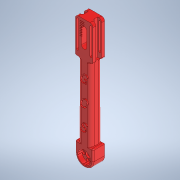
# Autodesk Inventor part: Eslabon1
Saved by Autodesk Inventor 2021 (Build 250183000, 183)
## iProperties
Created: 2022-10-26
Part Number: Eslabon1
Material: Generic
Document SubType Name: Modeling
Designer: USUARIO
Density: 1 g/cm^3
Appearance: Light Red
Mass: 84.0555 g
Surface Area: 248.63 cm^2
Volume: 84.0555 cm^3
Author: USUARIO
Autodesk Inventor part; units mm, degrees
ref_plane "YZ Plane" through (0, 0, 0) normal (1, 0, 0) x (0, 1, 0)
ref_plane "XZ Plane" through (0, 0, 0) normal (0, 1, 0) x (-1, 0, 0)
ref_plane "XY Plane" through (0, 0, 0) normal (0, 0, 1) x (1, 0, 0)
sketch "Sketch1" plane through (0, 0, 0) normal (0, 0, 1) x (1, 0, 0)
  line L0 (0, 0) -> (0, 190) construction
  line L1 (15, 0) -> (15, 190)
  line L2 (-15, 190) -> (-15, 0)
  arc A0 (-15, 0) -> (15, 0) centre (0, 0) ccw
  arc A1 (15, 190) -> (-15, 190) centre (0, 190) ccw
  line L3 (-15, 175) -> (15, 175)
  line L4 (15, 175) -> (15, 200)
  line L5 (10, 205) -> (-10, 205)
  line L6 (-15, 200) -> (-15, 175)
  line L7 (-15, 175) -> (15, 205) construction
  line L8 (15, 175) -> (-15, 205) construction
  arc A2 (-10, 205) -> (-15, 200) centre (-10, 200) ccw
  arc A3 (15, 200) -> (10, 205) centre (10, 200) ccw
  point P0 (0, 95)
  point P1 (0, 205)
  dimension "d0" = 190
  dimension "d1" = 30
  dimension "d48" = 5
  dimension "d49" = 30
  dimension "d50" = 30
  constraints: 20 end point, 8 point on circle, 8 tangent, 4 centre point, 4 point on line, 3 midpoint, 3 parallel, 1 equal radius, 1 horizontal, 1 perpendicular, 1 vertical
  measures "d0" distance of L0.start L0.end
  measures "d1" diameter of A1
  measures "d48" radius of A2
  measures "d49" distance between parallel lines of L6 L4
  measures "d50" distance between parallel lines of L3 L5
extrude "Extrusion1" add sketch "Sketch1" along normal blind 20
sketch "Sketch2" plane through (0, 0, 20) normal (0, 0, 1) x (1, 0, 0)
  arc A0 (15, 185) -> (-15, 185) centre (0, 185) ccw projected
  arc A1 (-15, 0) -> (15, 0) centre (0, 0) ccw projected
  circle A2 centre (0, 0) radius 11
  dimension "d4" = 22
  constraints: 1 centre point, 1 coincident
  measures "d4" diameter of A2
extrude "Extrusion2" cut sketch "Sketch2" against normal blind 7
sketch "Sketch3" plane through (0, 0, 0) normal (0, 0, -1) x (-1, 0, 0)
  circle A0 centre (0, 0) radius 11 projected
  circle A1 centre (0, 0) radius 11
  circle A2 centre (0, 0) radius 2
  circle A3 centre (0, 0) radius 8 construction
  arc A4 (15, 185) -> (-15, 185) centre (0, 185) ccw construction
  circle A5 centre (0, 8) radius 1.5
  line L0 (0, 0) -> (0, 12.8172) construction
  circle A6 centre (-8, 0) radius 1.5
  circle A7 centre (0, -8) radius 1.5
  circle A8 centre (8, 0) radius 1.5
  circle A9 centre (0, 0) radius 5
  dimension "d9" = 16
  dimension "d7" = 22
  dimension "d8" = 4
  dimension "d10" = 3
  dimension "d13" = 360
  dimension "d15" = 10
  constraints: 7 centre point, 4 coincident, 2 end point, 1 point on line, 1 vertical, 1 vertical alignment, 11 other
  measures "d7" diameter of A1
  measures "d8" diameter of A2
  measures "d10" diameter of A5
  measures "d15" diameter of A9
extrude "Extrusion4" cut sketch "Sketch3" against normal through all contours A5 | A6 | A7 | A8
sketch "Sketch4" plane through (0, 0, 13) normal (0, 0, 1) x (1, 0, 0)
  circle A0 centre (-8, 0) radius 1.5 projected
  circle A1 centre (0, 0) radius 2 construction
  circle A2 centre (0, 0) radius 8 construction
  line L0 (-5, 1.7321) -> (-5, -1.7321)
  line L1 (-5, -1.7321) -> (-8, -3.4641)
  line L2 (-8, -3.4641) -> (-11, -1.7321)
  line L3 (-11, -1.7321) -> (-11, 1.7321)
  line L4 (-11, 1.7321) -> (-8, 3.4641)
  line L5 (-8, 3.4641) -> (-5, 1.7321)
  line L6 (-3.4641, -8) -> (-1.7321, -5)
  line L7 (-1.7321, -5) -> (1.7321, -5)
  line L8 (1.7321, -5) -> (3.4641, -8)
  line L9 (3.4641, -8) -> (1.7321, -11)
  line L10 (1.7321, -11) -> (-1.7321, -11)
  line L11 (-1.7321, -11) -> (-3.4641, -8)
  line L12 (8, -3.4641) -> (5, -1.7321)
  line L13 (5, -1.7321) -> (5, 1.7321)
  line L14 (5, 1.7321) -> (8, 3.4641)
  line L15 (8, 3.4641) -> (11, 1.7321)
  line L16 (11, 1.7321) -> (11, -1.7321)
  line L17 (11, -1.7321) -> (8, -3.4641)
  line L18 (3.4641, 8) -> (1.7321, 5)
  line L19 (1.7321, 5) -> (-1.7321, 5)
  line L20 (-1.7321, 5) -> (-3.4641, 8)
  line L21 (-3.4641, 8) -> (-1.7321, 11)
  line L22 (-1.7321, 11) -> (1.7321, 11)
  line L23 (1.7321, 11) -> (3.4641, 8)
  dimension "d20" = 6
  dimension "d23" = 360
  constraints: 48 end point, 3 coincident, 1 horizontal alignment, 1 vertical, 64 other
  measures "d20" distance between parallel lines of L3 L0
extrude "Extrusion5" cut sketch "Sketch4" along normal blind 8.175 and the other way blind 3.5
extrude "Extrusion6" cut sketch "Sketch3" against normal blind 2 contours A0 | A2 | A9
extrude "Extrusion7" cut sketch "Sketch3" against normal through all contours A2
sketch "Sketch5" plane through (0, 0, 13) normal (0, 0, 1) x (1, 0, 0)
  circle A0 centre (0, 0) radius 2 projected
  circle A1 centre (0, 0) radius 4.5
  dimension "d33" = 9
  constraints: 1 centre point, 1 coincident
  measures "d33" diameter of A1
extrude "Extrusion8" cut sketch "Sketch5" against normal blind 3
sketch "Sketch9" plane through (0, 0, 20) normal (0, 0, 1) x (1, 0, 0)
  line L0 (-15, 200) -> (-15, 0) projected
  arc A0 (-15, 0) -> (15, 0) centre (0, 0) ccw projected
  line L1 (15, 0) -> (15, 200) projected
  arc A1 (15, 200) -> (10, 205) centre (10, 200) ccw projected
  line L2 (10, 205) -> (-10, 205) projected
  arc A2 (-10, 205) -> (-15, 200) centre (-10, 200) ccw projected
  line L3 (10.8485, 1.8195) -> (11, 1.7321) projected
  line L4 (11, 1.7321) -> (11, -1.7321) projected
  line L5 (11, -1.7321) -> (10.8485, -1.8195) projected
  arc A3 (1.8195, -10.8485) -> (10.8485, -1.8195) centre (0, 0) ccw projected
  line L6 (1.8195, -10.8485) -> (1.7321, -11) projected
  line L7 (1.7321, -11) -> (-1.7321, -11) projected
  line L8 (-1.7321, -11) -> (-1.8195, -10.8485) projected
  arc A4 (-10.8485, -1.8195) -> (-1.8195, -10.8485) centre (0, 0) ccw projected
  line L9 (-10.8485, -1.8195) -> (-11, -1.7321) projected
  line L10 (-11, -1.7321) -> (-11, 1.7321) projected
  line L11 (-11, 1.7321) -> (-10.8485, 1.8195) projected
  arc A5 (-1.8195, 10.8485) -> (-10.8485, 1.8195) centre (0, 0) ccw projected
  line L12 (-1.8195, 10.8485) -> (-1.7321, 11) projected
  line L13 (-1.7321, 11) -> (1.7321, 11) projected
  line L14 (1.7321, 11) -> (1.8195, 10.8485) projected
  arc A6 (10.8485, 1.8195) -> (1.8195, 10.8485) centre (0, 0) ccw projected
  line L15 (10, 205) -> (-10, 205) projected
  circle A7 centre (0, 0) radius 2 projected
  line L16 (0, 205) -> (0, 0) construction
  line L17 (0, 190) -> (0, 165) construction
  line L18 (-4.5, 190) -> (-4.5, 165)
  line L19 (4.5, 165) -> (4.5, 190)
  arc A8 (4.5, 190) -> (-4.5, 190) centre (0, 190) ccw
  arc A9 (-4.5, 165) -> (4.5, 165) centre (0, 165) ccw
  point P0 (0, 177.5)
  dimension "d51" = 25
  dimension "d52" = 9
  dimension "d53" = 190
  constraints: 10 end point, 4 point on circle, 4 tangent, 2 centre point, 2 midpoint, 2 point on line, 1 parallel, 1 vertical
  measures "d51" distance of L17.start L17.end
  measures "d52" diameter of A9
  measures "d53" distance of point (0, 0) L17.start
extrude "Extrusion11" cut sketch "Sketch9" against normal through all contours A8 L19 A9 L18
sketch "Sketch10" plane through (-10, 205, 0) normal (0, 1, 0) x (1, 0, 0)
  line L0 (14.5, -20) -> (5.5, -20) projected
  line L1 (5.5, -20) -> (14.5, -20) projected
  line L2 (-5, -20) -> (25, -20) projected
  line L3 (25, -20) -> (20, -20) projected
  line L4 (20, -20) -> (0, -20) projected
  line L5 (0, -20) -> (-5, -20) projected
  line L6 (20.8485, -20) -> (21, -20) projected
  line L7 (21, -20) -> (20.8485, -20) projected
  line L8 (20.8485, -20) -> (11.8195, -20) projected
  line L9 (11.8195, -20) -> (11.7321, -20) projected
  line L10 (11.7321, -20) -> (8.2679, -20) projected
  line L11 (8.2679, -20) -> (8.1805, -20) projected
  line L12 (8.1805, -20) -> (-0.8485, -20) projected
  line L13 (-0.8485, -20) -> (-1, -20) projected
  line L14 (-1, -20) -> (-0.8485, -20) projected
  line L15 (-0.8485, -20) -> (8.1805, -20) projected
  line L16 (8.1805, -20) -> (8.2679, -20) projected
  line L17 (8.2679, -20) -> (11.7321, -20) projected
  line L18 (11.7321, -20) -> (11.8195, -20) projected
  line L19 (11.8195, -20) -> (20.8485, -20) projected
  line L20 (25, 0) -> (25, -20) projected
  line L21 (25, 0) -> (25, -20) projected
  line L22 (14.5, 0) -> (5.5, 0) projected
  line L23 (5.5, 0) -> (14.5, 0) projected
  line L24 (-1, 0) -> (21, 0) projected
  line L25 (0, 0) -> (-5, 0) projected
  line L26 (20, 0) -> (0, 0) projected
  line L27 (25, 0) -> (20, 0) projected
  line L28 (-5, 0) -> (25, 0) projected
  line L29 (-5, 0) -> (-5, -20) projected
  line L30 (-5, 0) -> (-5, -20) projected
  line L31 (-5, 0) -> (-5, -20) projected
  line L32 (-5, -5) -> (2, -5)
  line L33 (2, -5) -> (2, -15)
  line L34 (2, -15) -> (-5, -15)
  line L35 (-5, -15) -> (-5, -5)
  line L36 (10, 0) -> (10, -20)
  line L37 (-5, -20) -> (25, -20) projected
  line L38 (25, -5) -> (18, -5)
  line L39 (18, -5) -> (18, -15)
  line L40 (18, -15) -> (25, -15)
  line L41 (25, -15) -> (25, -5)
  point P0 (-5, -15)
  dimension "d56" = 5
  dimension "d57" = 5
  dimension "d58" = 7
  constraints: 18 end point, 4 symmetric about line, 2 parallel, 1 horizontal, 1 perpendicular, 4 other
  measures "d56" distance between parallel lines of L28 L32
  measures "d57" distance between parallel lines of L2 L34
  measures "d58" distance of L33.end L34.end
extrude "Extrusion12" cut sketch "Sketch10" against normal blind 60 contours L40 L39 L38 L20 | L32 L33 L34 L29
sketch "Sketch11" plane through (0, 0, 0) normal (0, 0, -1) x (-1, 0, 0)
  arc A0 (-10, 205) -> (-15, 200) centre (-10, 200) ccw projected
  line L0 (-15, 145) -> (-15, 200) projected
  line L1 (-15, 145) -> (-8, 145) projected
  line L2 (-8, 205) -> (-8, 145) projected
  line L3 (-10, 205) -> (-8, 205) projected
  arc A1 (15, 200) -> (10, 205) centre (10, 200) ccw projected
  line L4 (8, 205) -> (10, 205) projected
  line L5 (8, 205) -> (8, 145) projected
  line L6 (8, 145) -> (15, 145) projected
  line L7 (15, 200) -> (15, 145) projected
  line L8 (-11.5, 145) -> (-11.5, 208.2052) construction
  line L9 (-11.5, 200) -> (-11.5, 155) construction
  line L10 (-13, 200) -> (-13, 155)
  line L11 (-10, 155) -> (-10, 200)
  arc A2 (-10, 200) -> (-13, 200) centre (-11.5, 200) ccw
  arc A3 (-13, 155) -> (-10, 155) centre (-11.5, 155) ccw
  arc A4 (-4.5, 165) -> (4.5, 165) centre (0, 165) ccw projected
  line L12 (4.5, 190) -> (4.5, 165) projected
  line L13 (-4.5, 165) -> (-4.5, 190) construction
  line L14 (-4.5, 177.5) -> (-11.5, 177.5) construction
  line L15 (-10, 205) -> (10, 205) projected
  line L16 (0, 205) -> (0, 150.8166) construction
  line L17 (13, 200) -> (13, 155)
  line L18 (10, 155) -> (10, 200)
  arc A5 (13, 200) -> (10, 200) centre (11.5, 200) ccw
  arc A6 (10, 155) -> (13, 155) centre (11.5, 155) ccw
  point P0 (0, 0)
  dimension "d61" = 3
  dimension "d62" = 45
  dimension "d73" = 23
  constraints: 18 end point, 8 point on circle, 6 symmetric about line, 4 centre point, 4 midpoint, 4 tangent, 2 point on line, 2 vertical, 1 horizontal, 1 parallel, 2 other
  measures "d61" diameter of A3
  measures "d62" distance of L10.start L10.end
  measures "d73" distance of A5.centre L9.start
extrude "Extrusion13" cut sketch "Sketch11" against normal through all contours A2 L11 A3 L10 | L17 A6 L18 A5
fillet "Fillet1" radius 4 2 edges at (8, 175, 15) (-8, 175, 15)
sketch "Sketch12" plane through (0, 0, 20) normal (0, 0, 1) x (1, 0, 0)
  line L0 (-19.28, 124.6729) -> (14.3731, 124.6729) construction
  line L1 (14.3731, 124.6729) -> (14.3731, 20.6875) construction
  line L2 (14.3731, 20.6875) -> (-19.28, 20.6875) construction
  line L3 (-19.28, 20.6875) -> (-19.28, 124.6729) construction
  line L4 (7.1676, 120.3037) -> (4.9576, 119.8084)
  spline S0 degree 2 poles (4.9576, 119.8084) (5.2116, 122.8566) (2.5952, 122.8566) knots 0 0 0 1 1 1
  spline S1 degree 2 poles (2.5952, 122.8566) (0.6138, 122.8566) (-1.0754, 121.1674) knots 0 0 0 1 1 1
  spline S2 degree 2 poles (-1.0754, 121.1674) (-2.6376, 119.6051) (-3.5521, 116.9252) knots 0 0 0 1 1 1
  spline S3 degree 2 poles (-3.5521, 116.9252) (-4.5936, 113.8261) (-3.8569, 112.2766) knots 0 0 0 1 1 1
  spline S4 degree 2 poles (-3.8569, 112.2766) (-3.2346, 110.9684) (-1.4691, 110.9684) knots 0 0 0 1 1 1
  spline S5 degree 2 poles (-1.4691, 110.9684) (0.2709, 110.9684) (1.7188, 112.4544) knots 0 0 0 1 1 1
  spline S6 degree 2 poles (1.7188, 112.4544) (2.9, 113.6737) (3.5478, 115.3757) knots 0 0 0 1 1 1
  line L5 (3.5478, 115.3757) -> (-0.3133, 115.3757)
  line L6 (-0.3133, 115.3757) -> (0.2963, 117.1665)
  line L7 (0.2963, 117.1665) -> (6.1896, 117.1665)
  line L8 (6.1896, 117.1665) -> (3.5351, 109.368)
  line L9 (3.5351, 109.368) -> (1.9348, 109.368)
  line L10 (1.9348, 109.368) -> (2.5825, 111.705)
  spline S7 degree 2 poles (2.5825, 111.705) (1.8332, 110.4476) (0.3852, 109.7491) knots 0 0 0 1 1 1
  spline S8 degree 2 poles (0.3852, 109.7491) (-0.8849, 109.1394) (-2.2312, 109.1394) knots 0 0 0 1 1 1
  spline S9 degree 2 poles (-2.2312, 109.1394) (-5.216, 109.1394) (-6.1177, 111.451) knots 0 0 0 1 1 1
  spline S10 degree 2 poles (-6.1177, 111.451) (-6.9306, 113.5213) (-5.7748, 116.8998) knots 0 0 0 1 1 1
  spline S11 degree 2 poles (-5.7748, 116.8998) (-4.4793, 120.7355) (-1.7232, 122.8693) knots 0 0 0 1 1 1
  spline S12 degree 2 poles (-1.7232, 122.8693) (0.6011, 124.6729) (3.1922, 124.6729) knots 0 0 0 1 1 1
  spline S13 degree 2 poles (3.1922, 124.6729) (5.4149, 124.6729) (6.1388, 123.4409) knots 0 0 0 1 1 1
  spline S14 degree 2 poles (6.1388, 123.4409) (7.3073, 122.2978) (7.1676, 120.3037) knots 0 0 0 1 1 1
  spline S15 degree 2 poles (2.9572, 88.3914) (5.942, 88.3914) (6.5262, 86.1687) knots 0 0 0 1 1 1
  spline S16 degree 2 poles (6.5262, 86.1687) (7.6947, 84.0095) (6.5516, 80.6564) knots 0 0 0 1 1 1
  spline S17 degree 2 poles (6.5516, 80.6564) (5.2434, 76.808) (2.5254, 74.6615) knots 0 0 0 1 1 1
  spline S18 degree 2 poles (2.5254, 74.6615) (0.2392, 72.8579) (-2.3265, 72.8579) knots 0 0 0 1 1 1
  spline S19 degree 2 poles (-2.3265, 72.8579) (-5.3112, 72.8579) (-6.2384, 75.1822) knots 0 0 0 1 1 1
  spline S20 degree 2 poles (-6.2384, 75.1822) (-7.0513, 77.2525) (-5.9209, 80.6056) knots 0 0 0 1 1 1
  spline S21 degree 2 poles (-5.9209, 80.6056) (-4.6, 84.454) (-1.8946, 86.5878) knots 0 0 0 1 1 1
  spline S22 degree 2 poles (-1.8946, 86.5878) (0.3916, 88.3914) (2.9572, 88.3914) knots 0 0 0 1 1 1
  spline S23 degree 2 poles (2.3348, 86.5751) (0.4043, 86.5751) (-1.0945, 85.2161) knots 0 0 0 1 1 1
  spline S24 degree 2 poles (-1.0945, 85.2161) (-2.7583, 83.3363) (-3.6855, 80.6437) knots 0 0 0 1 1 1
  spline S25 degree 2 poles (-3.6855, 80.6437) (-4.727, 77.5573) (-3.9903, 75.9824) knots 0 0 0 1 1 1
  spline S26 degree 2 poles (-3.9903, 75.9824) (-3.3806, 74.6869) (-1.7041, 74.6869) knots 0 0 0 1 1 1
  spline S27 degree 2 poles (-1.7041, 74.6869) (0.2392, 74.6869) (1.7379, 76.0713) knots 0 0 0 1 1 1
  spline S28 degree 2 poles (1.7379, 76.0713) (3.4017, 77.9384) (4.3162, 80.6437) knots 0 0 0 1 1 1
  spline S29 degree 2 poles (4.3162, 80.6437) (5.3704, 83.7301) (4.6337, 85.2923) knots 0 0 0 1 1 1
  spline S30 degree 2 poles (4.6337, 85.2923) (4.0241, 86.5751) (2.3348, 86.5751) knots 0 0 0 1 1 1
  line L11 (6.323, 48.3122) -> (4.0495, 47.728)
  spline S31 degree 2 poles (4.0495, 47.728) (4.1765, 50.319) (1.9792, 50.319) knots 0 0 0 1 1 1
  spline S32 degree 2 poles (1.9792, 50.319) (0.6075, 50.319) (-0.3578, 49.6459) knots 0 0 0 1 1 1
  spline S33 degree 2 poles (-0.3578, 49.6459) (-1.1707, 49.0743) (-1.4882, 48.1598) knots 0 0 0 1 1 1
  spline S34 degree 2 poles (-1.4882, 48.1598) (-1.8692, 47.0167) (-1.3866, 46.4579) knots 0 0 0 1 1 1
  spline S35 degree 2 poles (-1.3866, 46.4579) (-0.9293, 45.9371) (0.4932, 45.5561) knots 0 0 0 1 1 1
  line L12 (0.4932, 45.5561) -> (1.052, 45.3783)
  spline S36 degree 2 poles (1.052, 45.3783) (3.5796, 44.667) (4.1003, 43.1683) knots 0 0 0 1 1 1
  spline S37 degree 2 poles (4.1003, 43.1683) (4.6337, 42.5459) (4.0876, 40.9329) knots 0 0 0 1 1 1
  spline S38 degree 2 poles (4.0876, 40.9329) (3.3636, 38.8118) (1.0774, 37.5798) knots 0 0 0 1 1 1
  spline S39 degree 2 poles (1.0774, 37.5798) (-0.3324, 36.5764) (-2.6313, 36.5764) knots 0 0 0 1 1 1
  spline S40 degree 2 poles (-2.6313, 36.5764) (-4.8794, 36.5764) (-5.9336, 37.6687) knots 0 0 0 1 1 1
  spline S41 degree 2 poles (-5.9336, 37.6687) (-6.8862, 38.6467) (-6.7464, 40.5646) knots 0 0 0 1 1 1
  line L13 (-6.7464, 40.5646) -> (-4.4602, 41.2504)
  spline S42 degree 2 poles (-4.4602, 41.2504) (-4.6, 39.6628) (-3.7871, 38.8372) knots 0 0 0 1 1 1
  spline S43 degree 2 poles (-3.7871, 38.8372) (-3.2028, 38.3673) (-2.0597, 38.3673) knots 0 0 0 1 1 1
  spline S44 degree 2 poles (-2.0597, 38.3673) (-0.3832, 38.3673) (0.671, 39.1293) knots 0 0 0 1 1 1
  spline S45 degree 2 poles (0.671, 39.1293) (1.5093, 39.7263) (1.8522, 40.7424) knots 0 0 0 1 1 1
  spline S46 degree 2 poles (1.8522, 40.7424) (2.2459, 41.8982) (1.776, 42.4443) knots 0 0 0 1 1 1
  spline S47 degree 2 poles (1.776, 42.4443) (1.3061, 43.0286) (-0.3705, 43.5112) knots 0 0 0 1 1 1
  line L14 (-0.3705, 43.5112) -> (-0.9039, 43.689)
  spline S48 degree 2 poles (-0.9039, 43.689) (-3.1393, 44.3622) (-3.6474, 45.8228) knots 0 0 0 1 1 1
  spline S49 degree 2 poles (-3.6474, 45.8228) (-4.1935, 46.4452) (-3.6347, 48.0836) knots 0 0 0 1 1 1
  spline S50 degree 2 poles (-3.6347, 48.0836) (-3.025, 49.8999) (-1.2215, 51.043) knots 0 0 0 1 1 1
  spline S51 degree 2 poles (-1.2215, 51.043) (0.4551, 52.1099) (2.5508, 52.1099) knots 0 0 0 1 1 1
  spline S52 degree 2 poles (2.5508, 52.1099) (6.4373, 52.1099) (6.323, 48.3122) knots 0 0 0 1 1 1
  point P0 (0, 0)
  constraints: 2 other
extrude "Extrusion14" cut sketch "Sketch12" against normal blind 3
sketch "Sketch15" plane through (0, 0, 20) normal (0, 0, 1) x (1, 0, 0)
  line L0 (-11, 145.5) -> (11, 145.5)
  line L1 (11, 145.5) -> (11, 19)
  line L2 (11, 19) -> (-11, 19)
  line L3 (-11, 19) -> (-11, 145.5)
  line L4 (-15, 200) -> (-15, 0) projected
  line L5 (15, 0) -> (15, 200) projected
  arc A0 (10, 155) -> (13, 155) centre (11.5, 155) ccw projected
  line L6 (-1.7321, 11) -> (1.7321, 11) projected
  line L7 (-11, 145.5) -> (-15, 145.5)
  line L8 (-15, 145) -> (-15, 200) projected
  line L9 (11, 145.5) -> (15, 145.5)
  line L10 (15, 0) -> (15, 200) projected
  line L11 (11, 19) -> (15, 19)
  line L12 (-11, 19) -> (-15, 19)
  point P0 (0, 0)
  point P1 (-15, 145.5)
  point P2 (15, 145.5)
  dimension "d74" = 4
  dimension "d75" = 4
  dimension "d76" = 8
  dimension "d77" = 8
  constraints: 16 end point, 6 point on line, 2 horizontal, 2 parallel, 2 perpendicular
  measures "d74" distance between parallel lines of L4 L3
  measures "d75" distance between parallel lines of L5 L1
  measures "d76" distance edge to line of A0 L0
  measures "d77" distance between parallel lines of L6 L2
extrude "Extrusion15" cut sketch "Sketch15" against normal through all contours L3 L12 L4 L7 | L9 L5 L11 L1
fillet "Fillet2" radius 6 4 edges at (11, 82.25, 20) (11, 82.25, 0) (-11, 82.25, 20) (-11, 82.25, 0)
fillet "Fillet3" radius 2.6667 4 edges at (8.9281, 145.5, 18.5354) (-8.9281, 145.5, 18.5354) (8.873, 145.5, 1.4174) (-8.873, 145.5, 1.4174)
fillet "Fillet4" radius 2 4 edges at (-15, 145.5, 17.5) (15, 145.5, 17.5) (15, 145.5, 2.5) (-15, 145.5, 2.5)
fillet "Fillet5" radius 2 9 edges at (15, 19, 10) (10, 19, 20) (10, 19, 0) (-10, 19, 20) (-15, 19, 10) (-10, 19, 0) (0, -15, 20) (15, 9.5, 20) (-15, 9.5, 20)
sketch "Sketch16" plane through (0, 0, 20) normal (0, 0, 1) x (1, 0, 0)
  line L0 (5, 142.8333) -> (5, 124.3813) projected
  line L1 (11.2539, 145.5) -> (13, 145.5) projected
  arc A0 (13, 145.5) -> (15, 147.5) centre (13, 147.5) ccw projected
  line L2 (15, 147.5) -> (15, 200) projected
  arc A1 (15, 200) -> (10, 205) centre (10, 200) ccw projected
  line L3 (10, 205) -> (-10, 205) projected
  arc A2 (-10, 205) -> (-15, 200) centre (-10, 200) ccw projected
  line L4 (-15, 200) -> (-15, 147.5) projected
  arc A3 (-15, 147.5) -> (-13, 145.5) centre (-13, 147.5) ccw projected
  line L5 (-11.2539, 145.5) -> (-13, 145.5) projected
  line L6 (-5, 17) -> (-5, 37.0146) projected
  line L7 (-13, 17) -> (-5, 17) projected
  line L8 (-13, 0) -> (-13, 17) projected
  arc A4 (-13, 0) -> (13, 0) centre (0, 0) ccw projected
  line L9 (13, 17) -> (13, 0) projected
  line L10 (5, 17) -> (13, 17) projected
  line L11 (10.8485, 1.8195) -> (11, 1.7321) projected
  line L12 (11, 1.7321) -> (11, -1.7321) projected
  line L13 (11, -1.7321) -> (10.8485, -1.8195) projected
  arc A5 (1.8195, -10.8485) -> (10.8485, -1.8195) centre (0, 0) ccw projected
  line L14 (1.8195, -10.8485) -> (1.7321, -11) projected
  line L15 (1.7321, -11) -> (-1.7321, -11) projected
  line L16 (-1.7321, -11) -> (-1.8195, -10.8485) projected
  arc A6 (-10.8485, -1.8195) -> (-1.8195, -10.8485) centre (0, 0) ccw projected
  line L17 (-10.8485, -1.8195) -> (-11, -1.7321) projected
  line L18 (-11, -1.7321) -> (-11, 1.7321) projected
  line L19 (-11, 1.7321) -> (-10.8485, 1.8195) projected
  arc A7 (-1.8195, 10.8485) -> (-10.8485, 1.8195) centre (0, 0) ccw projected
  line L20 (-1.8195, 10.8485) -> (-1.7321, 11) projected
  line L21 (-1.7321, 11) -> (1.7321, 11) projected
  line L22 (1.7321, 11) -> (1.8195, 10.8485) projected
  arc A8 (10.8485, 1.8195) -> (1.8195, 10.8485) centre (0, 0) ccw projected
  line L23 (4.5, 190) -> (4.5, 165) projected
  arc A9 (-4.5, 165) -> (4.5, 165) centre (0, 165) ccw projected
  line L24 (-4.5, 165) -> (-4.5, 190) projected
  arc A10 (4.5, 190) -> (-4.5, 190) centre (0, 190) ccw projected
  line L25 (10, 155) -> (10, 200) projected
  arc A11 (13, 200) -> (10, 200) centre (11.5, 200) ccw projected
  line L26 (13, 200) -> (13, 155) projected
  arc A12 (10, 155) -> (13, 155) centre (11.5, 155) ccw projected
  arc A13 (-10, 200) -> (-13, 200) centre (-11.5, 200) ccw projected
  line L27 (-10, 200) -> (-10, 155) projected
  arc A14 (-13, 155) -> (-10, 155) centre (-11.5, 155) ccw projected
  line L28 (-13, 155) -> (-13, 200) projected
  line L29 (5, 47.9723) -> (4.0495, 47.728) projected
  line L30 (0.4932, 45.5561) -> (1.052, 45.3783) projected
  line L31 (-5, 41.0885) -> (-4.4602, 41.2504) projected
  line L32 (-0.3705, 43.5112) -> (-0.9039, 43.689) projected
  line L33 (5, 119.8179) -> (4.9576, 119.8084) projected
  line L34 (3.5478, 115.3757) -> (-0.3133, 115.3757) projected
  line L35 (-0.3133, 115.3757) -> (0.2963, 117.1665) projected
  line L36 (0.2963, 117.1665) -> (5, 117.1665) projected
  line L37 (5, 113.6716) -> (3.5351, 109.368) projected
  line L38 (3.5351, 109.368) -> (1.9348, 109.368) projected
  line L39 (1.9348, 109.368) -> (2.5825, 111.705) projected
  line L40 (-0.25, 200) -> (-7.25, 200) construction
  line L41 (-0.25, 200.25) -> (-7.25, 200.25)
  line L42 (-7.25, 199.75) -> (-0.25, 199.75)
  arc A15 (-0.25, 199.75) -> (-0.25, 200.25) centre (-0.25, 200) ccw
  arc A16 (-7.25, 200.25) -> (-7.25, 199.75) centre (-7.25, 200) ccw
  line L43 (0, -59.2071) -> (0, 250.2426) projected
  line L44 (-0.25, 195.25) -> (-7.25, 195.25)
  arc A17 (-7.25, 195.25) -> (-7.25, 194.75) centre (-7.25, 195) ccw
  line L45 (-7.25, 194.75) -> (-0.25, 194.75)
  arc A18 (-0.25, 194.75) -> (-0.25, 195.25) centre (-0.25, 195) ccw
  line L46 (-0.25, 190.25) -> (-7.25, 190.25)
  arc A19 (-7.25, 190.25) -> (-7.25, 189.75) centre (-7.25, 190) ccw
  line L47 (-7.25, 189.75) -> (-0.25, 189.75)
  arc A20 (-0.25, 189.75) -> (-0.25, 190.25) centre (-0.25, 190) ccw
  line L48 (-0.25, 185.25) -> (-7.25, 185.25)
  arc A21 (-7.25, 185.25) -> (-7.25, 184.75) centre (-7.25, 185) ccw
  line L49 (-7.25, 184.75) -> (-0.25, 184.75)
  arc A22 (-0.25, 184.75) -> (-0.25, 185.25) centre (-0.25, 185) ccw
  line L50 (-0.25, 180.25) -> (-7.25, 180.25)
  arc A23 (-7.25, 180.25) -> (-7.25, 179.75) centre (-7.25, 180) ccw
  line L51 (-7.25, 179.75) -> (-0.25, 179.75)
  arc A24 (-0.25, 179.75) -> (-0.25, 180.25) centre (-0.25, 180) ccw
  line L52 (-0.25, 197.5) -> (-7.25, 197.5) construction
  line L53 (-0.25, 197.75) -> (-7.25, 197.75)
  line L54 (-7.25, 197.25) -> (-0.25, 197.25)
  arc A25 (-0.25, 197.25) -> (-0.25, 197.75) centre (-0.25, 197.5) ccw
  arc A26 (-7.25, 197.75) -> (-7.25, 197.25) centre (-7.25, 197.5) ccw
  line L55 (-0.25, 192.75) -> (-7.25, 192.75)
  arc A27 (-7.25, 192.75) -> (-7.25, 192.25) centre (-7.25, 192.5) ccw
  line L56 (-7.25, 192.25) -> (-0.25, 192.25)
  arc A28 (-0.25, 192.25) -> (-0.25, 192.75) centre (-0.25, 192.5) ccw
  line L57 (-0.25, 187.75) -> (-7.25, 187.75)
  arc A29 (-7.25, 187.75) -> (-7.25, 187.25) centre (-7.25, 187.5) ccw
  line L58 (-7.25, 187.25) -> (-0.25, 187.25)
  arc A30 (-0.25, 187.25) -> (-0.25, 187.75) centre (-0.25, 187.5) ccw
  line L59 (-0.25, 182.75) -> (-7.25, 182.75)
  arc A31 (-7.25, 182.75) -> (-7.25, 182.25) centre (-7.25, 182.5) ccw
  line L60 (-7.25, 182.25) -> (-0.25, 182.25)
  arc A32 (-0.25, 182.25) -> (-0.25, 182.75) centre (-0.25, 182.5) ccw
  line L61 (-0.25, 177.75) -> (-7.25, 177.75)
  arc A33 (-7.25, 177.75) -> (-7.25, 177.25) centre (-7.25, 177.5) ccw
  line L62 (-7.25, 177.25) -> (-0.25, 177.25)
  arc A34 (-0.25, 177.25) -> (-0.25, 177.75) centre (-0.25, 177.5) ccw
  line L63 (5, 119.8179) -> (5, 117.1665) projected
  line L64 (5, 47.9723) -> (5, 17) projected
  line L65 (-5, 41.0885) -> (-5, 73.5698) projected
  line L66 (5, 77.3987) -> (5, 51.5153) projected
  line L67 (-5, 82.7675) -> (-5, 109.9225) projected
  line L68 (5, 113.6716) -> (5, 88.0183) projected
  line L69 (-5, 118.7842) -> (-5, 142.8333) projected
  point P0 (-3.75, 200)
  point P1 (-3.75, 197.5)
  point P2 (-3.8971, 192.25)
  point P3 (-3.562, 192.75)
  point P4 (-4.5, 189.75)
  point P5 (-4.4931, 190.25)
  point P6 (-4.5, 187.25)
  point P7 (-4.5, 187.75)
  point P8 (-4.5, 184.75)
  point P9 (-4.5, 185.25)
  point P10 (-4.5, 182.25)
  point P11 (-4.5, 182.75)
  point P12 (-4.5, 179.75)
  point P13 (-4.5, 180.25)
  point P14 (-4.5, 177.25)
  point P15 (-4.5, 177.75)
  dimension "d84" = 7
  dimension "d85" = 0.5
  dimension "d86" = 10
  dimension "d89" = 5
  dimension "d94" = 7
  dimension "d95" = 0.5
  dimension "d96" = 7.5
  dimension "d99" = 5
  constraints: 48 end point, 40 point on circle, 20 centre point, 10 tangent, 2 midpoint, 2 parallel, 2 vertical, 1 horizontal, 1 perpendicular, 122 other
  measures "d84" distance of L40.start L40.end
  measures "d85" diameter of A16
  measures "d86" distance from line of A10.centre L40
  measures "d89" distance of L41.start L44.start
  measures "d94" distance of L52.start L52.end
  measures "d95" diameter of A26
  measures "d96" distance from line of A10.centre L52
  measures "d99" distance of L53.start L55.start
extrude "Extrusion16" cut sketch "Sketch16" against normal blind 1 contours A10 L56 A27 L55 | L62 A33 L61 L24 | A10 L24 L47 A19 L46 | L51 A23 L50 L24 | L58 A29 L57 L24 | L60 A31 L59 L24 | L49 A21 L48 L24 | A15 L42 A16 L41 | A18 L45 A17 L44 | A25 L54 A26 L53
equation "\"d0\" = L1"
equation "\"d1\" = B1"
equation "\"d49\" = B1"
equation "\"d50\" = d49"
equation "\"d2\" = H1"
equation "\"d4\" = DER"
equation "\"d5\" = HR"
equation "\"d7\" = DER"
equation "\"d8\" = DEM"
equation "\"d53\" = Dmax"
equation "\"d57\" = d56"
equation "\"d74\" = RC"
equation "\"d75\" = RC"
equation "\"d76\" = 2 * RC"
equation "\"d77\" = 2 * RC"
equation "\"d80\" = 1.5 * RC"
equation "\"d81\" = 0.666667 * RC"
equation "\"L1\" = 190"
equation "\"B1\" = 30"
equation "\"H1\" = 20"
equation "\"DER\" = 22"
equation "\"DIR\" = 8"
equation "\"HR\" = 7"
equation "\"DEM\" = 4"
equation "\"Dmax\" = 190"
equation "\"Bsm\" = 22.5"
equation "\"Dmarc\" = 17.5"
equation "\"Hsm\" = 12"
equation "\"Dsc\" = 5"
equation "\"Lsm\" = 21"
equation "\"RC\" = 4"
equation "\"TB\" = 3"
equation "\"HSE\" = 25"
equation "\"PB\" = 25"
equation "\"LMaSP\" = 46.5"
body "Solid1"
